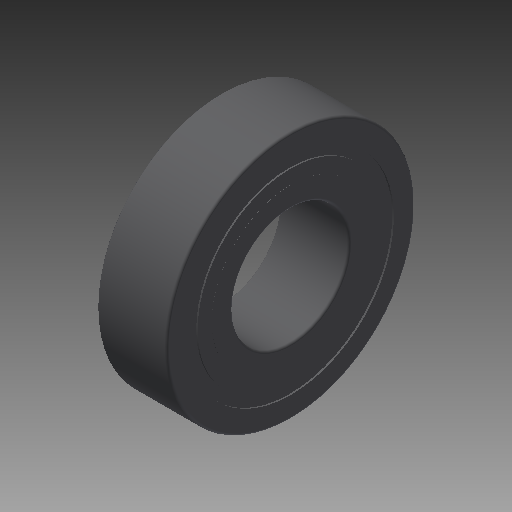
# Autodesk Inventor part: BF 15 Part2
Saved by Autodesk Inventor 2018 (Build 220112000, 112)
## iProperties
Category: PARTsolutions
Company: THK
Created: 2017-05-30
Part Number: BF 15 Part2
Catalog Web Link: www.cadenas.de
Description: Supported side type BF-P2-
Vendor: THK
Document SubType Name: Modeling
Designer: psAdmin
Manufacturer: THK
Mass: 5.59741 g
Surface Area: 26.0894 cm^2
Volume: 5.59741 cm^3
Density: 1 g/cm^3
Material: Generic
Appearance: PSOLRGB-192-192-192
PSOL_IDENT_0: {$CADENAS_DATA\23d-libs\thk\fed_screw\ball_screw\ball_screw_peripheral\suport_unit\supported_bf_2.pr
PSOL_IDENT_1: j},183 {VTYP=3D},{NB=BF 15 Part2},{LINA=BF 15 Part2},{NN=Supported side type BF-P2},{DATE=16.05.2017
PSOL_IDENT_2: 06:09:50},{GEOMDATE=02.02.2010 00:00:00},{VERSION=},{LINEID=30},{LINESUBID=-1},{WBVAR=}  {NB=BF 15
PSOL_IDENT_3: Part2},{LINA=BF 15 Part2},{KT=DUMMY},{IDNR=},{MN=BF 15},{SDX=32.000},{LX=9.000},{SD=15.000},{D1=26.5
PSOL_IDENT_4: 00},{D2=24.000},{D3=20.400}
NN: Supported side type BF-P2
NB: BF 15 Part2
NBSYN: $MN. Part2
LINA: BF 15 Part2
MN: BF 15
SDX: 32.000
LX: 9.000
SD: 15.000
D1: 26.500
D2: 24.000
D3: 20.400
SUPPLIER: THK
ARTICLENO: BF 15 Part2
BOMINFO: BF 15 Part2
CREATOR: CADENAS GmbH
Title: BF 15 Part2
Author: Cadenas PARTsolutions
Autodesk Inventor part; units mm, degrees
sketch "Sketch_1" plane through (0, 0, 0) normal (0, 0, 1) x (1, 0, 0)
  line L0 (50, 0) -> (-50, 0)
  arc A0 (-4.5, 7.8) -> (-4.2, 7.5) centre (-4.2, 7.8) ccw
  line L1 (-4.2, 7.5) -> (4.2, 7.5)
  arc A1 (4.2, 7.5) -> (4.5, 7.8) centre (4.2, 7.8) ccw
  line L2 (4.5, 7.8) -> (4.5, 15.7)
  arc A2 (4.5, 15.7) -> (4.2, 16) centre (4.2, 15.7) ccw
  line L3 (4.2, 16) -> (-4.2, 16)
  arc A3 (-4.2, 16) -> (-4.5, 15.7) centre (-4.2, 15.7) ccw
  line L4 (-4.5, 15.7) -> (-4.5, 7.8)
  constraints: 10 end point, 8 point on circle, 4 centre point
revolve "Revolution1" add sketch "Sketch_1" angle 360 about axis through (50, 0, 0) along (1, 0, 0)
sketch "Sketch_2" plane through (0, 0, 0) normal (0, 0, 1) x (1, 0, 0)
  line L0 (50, 0) -> (-50, 0)
  line L1 (-6.3, 13.25) -> (-6.3, 7.5)
  line L2 (-6.3, 7.5) -> (-4.5, 7.5)
  line L3 (-4.5, 7.5) -> (-4.5, 10.2)
  line L4 (-4.5, 10.2) -> (-4.48, 10.2)
  line L5 (-4.48, 10.2) -> (-4.48, 12)
  line L6 (-4.48, 12) -> (-4.3, 12)
  line L7 (-4.3, 12) -> (-4.3, 13.25)
  line L8 (-4.3, 13.25) -> (-6.3, 13.25)
  constraints: 18 end point
revolve "Revolution2" cut sketch "Sketch_2" angle 360 about axis through (50, 0, 0) along (1, 0, 0)
sketch "Sketch_3" plane through (0, 0, 0) normal (0, 0, 1) x (1, 0, 0)
  line L0 (50, 0) -> (-50, 0)
  line L1 (4.3, 12) -> (4.48, 12)
  line L2 (4.48, 12) -> (4.48, 10.2)
  line L3 (4.48, 10.2) -> (4.5, 10.2)
  line L4 (4.5, 10.2) -> (4.5, 7.5)
  line L5 (4.5, 7.5) -> (6.3, 7.5)
  line L6 (6.3, 7.5) -> (6.3, 13.25)
  line L7 (6.3, 13.25) -> (4.3, 13.25)
  line L8 (4.3, 13.25) -> (4.3, 12)
  constraints: 18 end point
revolve "Revolution3" cut sketch "Sketch_3" angle 360 about axis through (50, 0, 0) along (1, 0, 0)
ref_plane "bf_2_XY" through (0, 0, 0) normal (1, 0, 0) x (0, 0, -1)
ref_plane "bf_2_YZ" through (0, 0, 0) normal (0, 0, -1) x (0, 1, 0)
ref_plane "bf_2_ZX" through (0, 0, 0) normal (0, 1, 0) x (1, 0, 0)
body "Solid1"
